Autodesk Inventor part; units mm, degrees
(part 2 of 2)
sketch "Sketch6" plane through (0.198, 6.7657, 76.2) normal (0.8660254, 0.5, 0) x (0, 0, -1)
  line L0 (9.5837, -3.7706) -> (68.3434, -3.7706) construction
  line L1 (68.3434, -3.7706) -> (68.3434, -8.4681) construction
  line L2 (68.3434, -8.4681) -> (9.5837, -8.4681) construction
  line L3 (9.5837, -8.4681) -> (9.5837, -3.7706) construction
  spline S0 degree 2 poles (10.7422, -7.0088) (10.4112, -7.0088) (9.9468, -6.8705) (9.7418, -6.7717) knots 0 0 0 1 2 2 2
  line L4 (9.7418, -6.7717) -> (9.7418, -6.2629)
  line L5 (9.7418, -6.2629) -> (9.7715, -6.2629)
  spline S1 degree 2 poles (9.7715, -6.2629) (9.9715, -6.4506) (10.4779, -6.6581) (10.7125, -6.6581) knots 0 0 0 1 2 2 2
  spline S2 degree 2 poles (10.7125, -6.6581) (11.0485, -6.6581) (11.3918, -6.379) (11.3918, -6.1492) knots 0 0 0 1 2 2 2
  spline S3 degree 2 poles (11.3918, -6.1492) (11.3918, -5.9665) (11.2115, -5.7392) (11.0164, -5.6824) knots 0 0 0 1 2 2 2
  spline S4 degree 2 poles (11.0164, -5.6824) (10.8756, -5.6429) (10.6409, -5.5886) (10.4655, -5.5441) knots 0 0 0 1 2 2 2
  spline S5 degree 2 poles (10.4655, -5.5441) (10.3075, -5.5021) (10.058, -5.3761) (9.9617, -5.2749) knots 0 0 0 1 2 2 2
  spline S6 degree 2 poles (9.9617, -5.2749) (9.8678, -5.1736) (9.7641, -4.9019) (9.7641, -4.724) knots 0 0 0 1 2 2 2
  spline S7 degree 2 poles (9.7641, -4.724) (9.7641, -4.3535) (10.342, -3.8521) (10.7891, -3.8521) knots 0 0 0 1 2 2 2
  spline S8 degree 2 poles (10.7891, -3.8521) (11.046, -3.8521) (11.5005, -3.9534) (11.6956, -4.0497) knots 0 0 0 1 2 2 2
  line L6 (11.6956, -4.0497) -> (11.6956, -4.5339)
  line L7 (11.6956, -4.5339) -> (11.666, -4.5339)
  spline S9 degree 2 poles (11.666, -4.5339) (11.5202, -4.4005) (11.0658, -4.2029) (10.8163, -4.2029) knots 0 0 0 1 2 2 2
  spline S10 degree 2 poles (10.8163, -4.2029) (10.5347, -4.2029) (10.1864, -4.4672) (10.1864, -4.6821) knots 0 0 0 1 2 2 2
  spline S11 degree 2 poles (10.1864, -4.6821) (10.1864, -4.8747) (10.3914, -5.1044) (10.5841, -5.1563) knots 0 0 0 1 2 2 2
  spline S12 degree 2 poles (10.5841, -5.1563) (10.7125, -5.1909) (11.0855, -5.2798) (11.209, -5.3169) knots 0 0 0 1 2 2 2
  spline S13 degree 2 poles (11.209, -5.3169) (11.5227, -5.4132) (11.8142, -5.801) (11.8142, -6.085) knots 0 0 0 1 2 2 2
  spline S14 degree 2 poles (11.8142, -6.085) (11.8142, -6.2653) (11.6684, -6.6111) (11.5375, -6.7322) knots 0 0 0 1 2 2 2
  spline S15 degree 2 poles (11.5375, -6.7322) (11.3918, -6.8656) (11.0213, -7.0088) (10.7422, -7.0088) knots 0 0 0 1 2 2 2
  spline S16 degree 2 poles (14.0767, -5.8109) (14.0767, -6.3888) (13.521, -7.0187) (13.0566, -7.0187) knots 0 0 0 1 2 2 2
  spline S17 degree 2 poles (13.0566, -7.0187) (12.5799, -7.0187) (12.034, -6.3691) (12.034, -5.8109) knots 0 0 0 1 2 2 2
  spline S18 degree 2 poles (12.034, -5.8109) (12.034, -5.2378) (12.5972, -4.603) (13.0566, -4.603) knots 0 0 0 1 2 2 2
  spline S19 degree 2 poles (13.0566, -4.603) (13.521, -4.603) (14.0767, -5.2353) (14.0767, -5.8109) knots 0 0 0 1 2 2 2
  spline S20 degree 2 poles (13.679, -5.8109) (13.679, -5.3663) (13.3555, -4.934) (13.0566, -4.934) knots 0 0 0 1 2 2 2
  spline S21 degree 2 poles (13.0566, -4.934) (12.7577, -4.934) (12.4317, -5.3663) (12.4317, -5.8109) knots 0 0 0 1 2 2 2
  spline S22 degree 2 poles (12.4317, -5.8109) (12.4317, -6.2431) (12.7577, -6.6877) (13.0566, -6.6877) knots 0 0 0 1 2 2 2
  spline S23 degree 2 poles (13.0566, -6.6877) (13.353, -6.6877) (13.679, -6.2505) (13.679, -5.8109) knots 0 0 0 1 2 2 2
  line L8 (17.0654, -6.9545) -> (17.0654, -5.6305)
  spline S24 degree 2 poles (17.0654, -5.6305) (17.0654, -5.4725) (17.0407, -5.2032) (17.0012, -5.1291) knots 0 0 0 1 2 2 2
  spline S25 degree 2 poles (17.0012, -5.1291) (16.9617, -5.0476) (16.811, -4.9686) (16.6801, -4.9686) knots 0 0 0 1 2 2 2
  spline S26 degree 2 poles (16.6801, -4.9686) (16.5615, -4.9686) (16.2898, -5.1143) (16.1466, -5.2526) knots 0 0 0 1 2 2 2
  spline S27 degree 2 poles (16.1466, -5.2526) (16.1491, -5.2872) (16.154, -5.3835) (16.154, -5.4478) knots 0 0 0 1 2 2 2
  line L9 (16.154, -5.4478) -> (16.154, -6.9545)
  line L10 (16.154, -6.9545) -> (15.7687, -6.9545)
  line L11 (15.7687, -6.9545) -> (15.7687, -5.6305)
  spline S28 degree 2 poles (15.7687, -5.6305) (15.7687, -5.4725) (15.744, -5.2032) (15.7044, -5.1291) knots 0 0 0 1 2 2 2
  spline S29 degree 2 poles (15.7044, -5.1291) (15.6649, -5.0476) (15.5143, -4.9686) (15.3833, -4.9686) knots 0 0 0 1 2 2 2
  spline S30 degree 2 poles (15.3833, -4.9686) (15.2598, -4.9686) (14.9857, -5.1242) (14.8572, -5.2452) knots 0 0 0 1 2 2 2
  line L12 (14.8572, -5.2452) -> (14.8572, -6.9545)
  line L13 (14.8572, -6.9545) -> (14.4719, -6.9545)
  line L14 (14.4719, -6.9545) -> (14.4719, -4.6672)
  line L15 (14.4719, -4.6672) -> (14.8572, -4.6672)
  line L16 (14.8572, -4.6672) -> (14.8572, -4.9192)
  spline S31 degree 2 poles (14.8572, -4.9192) (15.0079, -4.7685) (15.3043, -4.603) (15.4821, -4.603) knots 0 0 0 1 2 2 2
  spline S32 degree 2 poles (15.4821, -4.603) (15.6847, -4.603) (15.9984, -4.7883) (16.0799, -4.9982) knots 0 0 0 1 2 2 2
  spline S33 degree 2 poles (16.0799, -4.9982) (16.2553, -4.8031) (16.5862, -4.603) (16.7789, -4.603) knots 0 0 0 1 2 2 2
  spline S34 degree 2 poles (16.7789, -4.603) (16.9271, -4.603) (17.1692, -4.6944) (17.2581, -4.7981) knots 0 0 0 1 2 2 2
  spline S35 degree 2 poles (17.2581, -4.7981) (17.3495, -4.9019) (17.4507, -5.2131) (17.4507, -5.4478) knots 0 0 0 1 2 2 2
  line L17 (17.4507, -5.4478) -> (17.4507, -6.9545)
  line L18 (17.4507, -6.9545) -> (17.0654, -6.9545)
  spline S36 degree 2 poles (18.9846, -7.0063) (18.4363, -7.0063) (17.8336, -6.3913) (17.8336, -5.8232) knots 0 0 0 1 2 2 2
  spline S37 degree 2 poles (17.8336, -5.8232) (17.8336, -5.265) (18.419, -4.603) (18.8908, -4.603) knots 0 0 0 1 2 2 2
  spline S38 degree 2 poles (18.8908, -4.603) (19.1032, -4.603) (19.4317, -4.7265) (19.5527, -4.8574) knots 0 0 0 1 2 2 2
  spline S39 degree 2 poles (19.5527, -4.8574) (19.6762, -4.9883) (19.8071, -5.3663) (19.8071, -5.6404) knots 0 0 0 1 2 2 2
  line L19 (19.8071, -5.6404) -> (19.8071, -5.8504)
  line L20 (19.8071, -5.8504) -> (18.2239, -5.8504)
  spline S40 degree 2 poles (18.2239, -5.8504) (18.2239, -6.248) (18.624, -6.6704) (18.9797, -6.6704) knots 0 0 0 1 2 2 2
  spline S41 degree 2 poles (18.9797, -6.6704) (19.1057, -6.6704) (19.3502, -6.6136) (19.449, -6.5691) knots 0 0 0 1 2 2 2
  spline S42 degree 2 poles (19.449, -6.5691) (19.5527, -6.5197) (19.696, -6.4333) (19.7429, -6.3938) knots 0 0 0 1 2 2 2
  line L21 (19.7429, -6.3938) -> (19.7652, -6.3938)
  line L22 (19.7652, -6.3938) -> (19.7652, -6.8137)
  spline S43 degree 2 poles (19.7652, -6.8137) (19.6985, -6.8409) (19.4959, -6.9199) (19.4169, -6.9421) knots 0 0 0 1 2 2 2
  spline S44 degree 2 poles (19.4169, -6.9421) (19.3057, -6.9742) (19.123, -7.0063) (18.9846, -7.0063) knots 0 0 0 1 2 2 2
  spline S45 degree 2 poles (19.4317, -5.5564) (19.4268, -5.4008) (19.3625, -5.1736) (19.3008, -5.097) knots 0 0 0 1 2 2 2
  spline S46 degree 2 poles (19.3008, -5.097) (19.2341, -5.0106) (19.0241, -4.9192) (18.8685, -4.9192) knots 0 0 0 1 2 2 2
  spline S47 degree 2 poles (18.8685, -4.9192) (18.7154, -4.9192) (18.5005, -5.0106) (18.4116, -5.0995) knots 0 0 0 1 2 2 2
  spline S48 degree 2 poles (18.4116, -5.0995) (18.3251, -5.1909) (18.2362, -5.4107) (18.2239, -5.5564) knots 0 0 0 1 2 2 2
  line L23 (18.2239, -5.5564) -> (19.4317, -5.5564)
  line L24 (23.895, -6.9545) -> (23.3689, -6.9545)
  line L25 (23.3689, -6.9545) -> (22.4056, -5.7417)
  line L26 (22.4056, -5.7417) -> (21.9412, -5.7417)
  line L27 (21.9412, -5.7417) -> (21.9412, -6.9545)
  line L28 (21.9412, -6.9545) -> (21.5362, -6.9545)
  line L29 (21.5362, -6.9545) -> (21.5362, -3.9065)
  line L30 (21.5362, -3.9065) -> (22.3216, -3.9065)
  spline S49 degree 2 poles (22.3216, -3.9065) (22.5834, -3.9065) (22.9367, -3.9633) (23.0972, -4.067) knots 0 0 0 1 2 2 2
  spline S50 degree 2 poles (23.0972, -4.067) (23.2578, -4.1708) (23.443, -4.4943) (23.443, -4.7339) knots 0 0 0 1 2 2 2
  spline S51 degree 2 poles (23.443, -4.7339) (23.443, -5.0674) (23.1021, -5.5194) (22.8107, -5.6281) knots 0 0 0 1 2 2 2
  line L31 (22.8107, -5.6281) -> (23.895, -6.9545)
  spline S52 degree 2 poles (23.0206, -4.766) (23.0206, -4.6327) (22.9268, -4.4276) (22.828, -4.361) knots 0 0 0 1 2 2 2
  spline S53 degree 2 poles (22.828, -4.361) (22.7415, -4.3041) (22.5118, -4.2572) (22.3439, -4.2572) knots 0 0 0 1 2 2 2
  line L32 (22.3439, -4.2572) -> (21.9412, -4.2572)
  line L33 (21.9412, -4.2572) -> (21.9412, -5.4033)
  line L34 (21.9412, -5.4033) -> (22.2969, -5.4033)
  spline S54 degree 2 poles (22.2969, -5.4033) (22.4723, -5.4033) (22.7514, -5.3416) (22.8477, -5.2452) knots 0 0 0 1 2 2 2
  spline S55 degree 2 poles (22.8477, -5.2452) (22.9367, -5.1612) (23.0206, -4.9241) (23.0206, -4.766) knots 0 0 0 1 2 2 2
  spline S56 degree 2 poles (25.382, -6.7124) (25.335, -6.747) (25.177, -6.8705) (25.1029, -6.9075) knots 0 0 0 1 2 2 2
  spline S57 degree 2 poles (25.1029, -6.9075) (25.0016, -6.9619) (24.8114, -7.0187) (24.6385, -7.0187) knots 0 0 0 1 2 2 2
  spline S58 degree 2 poles (24.6385, -7.0187) (24.4977, -7.0187) (24.2433, -6.9125) (24.147, -6.8162) knots 0 0 0 1 2 2 2
  spline S59 degree 2 poles (24.147, -6.8162) (24.0556, -6.7223) (23.9444, -6.4456) (23.9444, -6.2925) knots 0 0 0 1 2 2 2
  spline S60 degree 2 poles (23.9444, -6.2925) (23.9444, -6.0554) (24.1445, -5.7195) (24.3619, -5.6231) knots 0 0 0 1 2 2 2
  spline S61 degree 2 poles (24.3619, -5.6231) (24.5545, -5.5342) (25.0782, -5.4675) (25.382, -5.4502) knots 0 0 0 1 2 2 2
  line L35 (25.382, -5.4502) -> (25.382, -5.3761)
  spline S62 degree 2 poles (25.382, -5.3761) (25.382, -5.2428) (25.3005, -5.0773) (25.2264, -5.0303) knots 0 0 0 1 2 2 2
  spline S63 degree 2 poles (25.2264, -5.0303) (25.1523, -4.9834) (24.9398, -4.9538) (24.8262, -4.9538) knots 0 0 0 1 2 2 2
  spline S64 degree 2 poles (24.8262, -4.9538) (24.6928, -4.9538) (24.3322, -5.0328) (24.1519, -5.1094) knots 0 0 0 1 2 2 2
  line L36 (24.1519, -5.1094) -> (24.1297, -5.1094)
  line L37 (24.1297, -5.1094) -> (24.1297, -4.7166)
  spline S65 degree 2 poles (24.1297, -4.7166) (24.2359, -4.687) (24.6336, -4.6129) (24.8287, -4.6129) knots 0 0 0 1 2 2 2
  spline S66 degree 2 poles (24.8287, -4.6129) (25.0658, -4.6129) (25.3894, -4.687) (25.5178, -4.7833) knots 0 0 0 1 2 2 2
  spline S67 degree 2 poles (25.5178, -4.7833) (25.6438, -4.8772) (25.7673, -5.1761) (25.7673, -5.391) knots 0 0 0 1 2 2 2
  line L38 (25.7673, -5.391) -> (25.7673, -6.9545)
  line L39 (25.7673, -6.9545) -> (25.382, -6.9545)
  line L40 (25.382, -6.9545) -> (25.382, -6.7124)
  line L41 (25.382, -6.3913) -> (25.382, -5.7565)
  spline S68 degree 2 poles (25.382, -5.7565) (25.2437, -5.7689) (24.8262, -5.8109) (24.6953, -5.8504) knots 0 0 0 1 2 2 2
  spline S69 degree 2 poles (24.6953, -5.8504) (24.5422, -5.8973) (24.3421, -6.0924) (24.3421, -6.2653) knots 0 0 0 1 2 2 2
  spline S70 degree 2 poles (24.3421, -6.2653) (24.3421, -6.4629) (24.5644, -6.663) (24.7768, -6.663) knots 0 0 0 1 2 2 2
  spline S71 degree 2 poles (24.7768, -6.663) (24.9571, -6.663) (25.2535, -6.5074) (25.382, -6.3913) knots 0 0 0 1 2 2 2
  line L42 (28.1039, -6.9545) -> (27.7186, -6.9545)
  line L43 (27.7186, -6.9545) -> (27.7186, -5.6503)
  spline S72 degree 2 poles (27.7186, -5.6503) (27.7186, -5.4922) (27.689, -5.2205) (27.6445, -5.139) knots 0 0 0 1 2 2 2
  spline S73 degree 2 poles (27.6445, -5.139) (27.5976, -5.0526) (27.4296, -4.9686) (27.2864, -4.9686) knots 0 0 0 1 2 2 2
  spline S74 degree 2 poles (27.2864, -4.9686) (27.1431, -4.9686) (26.8393, -5.1217) (26.6935, -5.2452) knots 0 0 0 1 2 2 2
  line L44 (26.6935, -5.2452) -> (26.6935, -6.9545)
  line L45 (26.6935, -6.9545) -> (26.3082, -6.9545)
  line L46 (26.3082, -6.9545) -> (26.3082, -4.6672)
  line L47 (26.3082, -4.6672) -> (26.6935, -4.6672)
  line L48 (26.6935, -4.6672) -> (26.6935, -4.9216)
  spline S75 degree 2 poles (26.6935, -4.9216) (26.8665, -4.766) (27.1999, -4.603) (27.3876, -4.603) knots 0 0 0 1 2 2 2
  spline S76 degree 2 poles (27.3876, -4.603) (27.7235, -4.603) (28.1039, -5.0476) (28.1039, -5.47) knots 0 0 0 1 2 2 2
  line L49 (28.1039, -5.47) -> (28.1039, -6.9545)
  line L50 (30.4035, -6.9545) -> (30.0182, -6.9545)
  line L51 (30.0182, -6.9545) -> (30.0182, -6.7223)
  spline S77 degree 2 poles (30.0182, -6.7223) (29.9293, -6.7964) (29.7984, -6.8952) (29.7094, -6.9372) knots 0 0 0 1 2 2 2
  spline S78 degree 2 poles (29.7094, -6.9372) (29.6279, -6.9767) (29.4526, -7.0187) (29.3365, -7.0187) knots 0 0 0 1 2 2 2
  spline S79 degree 2 poles (29.3365, -7.0187) (29.1487, -7.0187) (28.8326, -6.8631) (28.7214, -6.7124) knots 0 0 0 1 2 2 2
  spline S80 degree 2 poles (28.7214, -6.7124) (28.6103, -6.5617) (28.4868, -6.1171) (28.4868, -5.8281) knots 0 0 0 1 2 2 2
  spline S81 degree 2 poles (28.4868, -5.8281) (28.4868, -5.5268) (28.6424, -5.0871) (28.7782, -4.9216) knots 0 0 0 1 2 2 2
  spline S82 degree 2 poles (28.7782, -4.9216) (28.9042, -4.7734) (29.2574, -4.603) (29.4526, -4.603) knots 0 0 0 1 2 2 2
  spline S83 degree 2 poles (29.4526, -4.603) (29.623, -4.603) (29.8774, -4.6796) (30.0182, -4.7586) knots 0 0 0 1 2 2 2
  line L52 (30.0182, -4.7586) -> (30.0182, -3.7706)
  line L53 (30.0182, -3.7706) -> (30.4035, -3.7706)
  line L54 (30.4035, -3.7706) -> (30.4035, -6.9545)
  line L55 (30.0182, -6.3987) -> (30.0182, -5.0773)
  spline S84 degree 2 poles (30.0182, -5.0773) (29.8749, -5.0081) (29.6477, -4.9562) (29.5168, -4.9562) knots 0 0 0 1 2 2 2
  spline S85 degree 2 poles (29.5168, -4.9562) (29.2204, -4.9562) (28.8845, -5.4008) (28.8845, -5.8207) knots 0 0 0 1 2 2 2
  spline S86 degree 2 poles (28.8845, -5.8207) (28.8845, -6.2258) (29.1413, -6.6531) (29.4254, -6.6531) knots 0 0 0 1 2 2 2
  spline S87 degree 2 poles (29.4254, -6.6531) (29.5761, -6.6531) (29.8823, -6.5148) (30.0182, -6.3987) knots 0 0 0 1 2 2 2
  spline S88 degree 2 poles (32.8414, -5.8109) (32.8414, -6.3888) (32.2857, -7.0187) (31.8213, -7.0187) knots 0 0 0 1 2 2 2
  spline S89 degree 2 poles (31.8213, -7.0187) (31.3446, -7.0187) (30.7987, -6.3691) (30.7987, -5.8109) knots 0 0 0 1 2 2 2
  spline S90 degree 2 poles (30.7987, -5.8109) (30.7987, -5.2378) (31.3619, -4.603) (31.8213, -4.603) knots 0 0 0 1 2 2 2
  spline S91 degree 2 poles (31.8213, -4.603) (32.2857, -4.603) (32.8414, -5.2353) (32.8414, -5.8109) knots 0 0 0 1 2 2 2
  spline S92 degree 2 poles (32.4437, -5.8109) (32.4437, -5.3663) (32.1202, -4.934) (31.8213, -4.934) knots 0 0 0 1 2 2 2
  spline S93 degree 2 poles (31.8213, -4.934) (31.5224, -4.934) (31.1964, -5.3663) (31.1964, -5.8109) knots 0 0 0 1 2 2 2
  spline S94 degree 2 poles (31.1964, -5.8109) (31.1964, -6.2431) (31.5224, -6.6877) (31.8213, -6.6877) knots 0 0 0 1 2 2 2
  spline S95 degree 2 poles (31.8213, -6.6877) (32.1177, -6.6877) (32.4437, -6.2505) (32.4437, -5.8109) knots 0 0 0 1 2 2 2
  line L56 (35.8301, -6.9545) -> (35.8301, -5.6305)
  spline S96 degree 2 poles (35.8301, -5.6305) (35.8301, -5.4725) (35.8054, -5.2032) (35.7659, -5.1291) knots 0 0 0 1 2 2 2
  spline S97 degree 2 poles (35.7659, -5.1291) (35.7264, -5.0476) (35.5757, -4.9686) (35.4448, -4.9686) knots 0 0 0 1 2 2 2
  spline S98 degree 2 poles (35.4448, -4.9686) (35.3263, -4.9686) (35.0546, -5.1143) (34.9113, -5.2526) knots 0 0 0 1 2 2 2
  spline S99 degree 2 poles (34.9113, -5.2526) (34.9138, -5.2872) (34.9187, -5.3835) (34.9187, -5.4478) knots 0 0 0 1 2 2 2
  line L57 (34.9187, -5.4478) -> (34.9187, -6.9545)
  line L58 (34.9187, -6.9545) -> (34.5334, -6.9545)
  line L59 (34.5334, -6.9545) -> (34.5334, -5.6305)
  spline S100 degree 2 poles (34.5334, -5.6305) (34.5334, -5.4725) (34.5087, -5.2032) (34.4692, -5.1291) knots 0 0 0 1 2 2 2
  spline S101 degree 2 poles (34.4692, -5.1291) (34.4296, -5.0476) (34.279, -4.9686) (34.1481, -4.9686) knots 0 0 0 1 2 2 2
  spline S102 degree 2 poles (34.1481, -4.9686) (34.0246, -4.9686) (33.7504, -5.1242) (33.6219, -5.2452) knots 0 0 0 1 2 2 2
  line L60 (33.6219, -5.2452) -> (33.6219, -6.9545)
  line L61 (33.6219, -6.9545) -> (33.2366, -6.9545)
  line L62 (33.2366, -6.9545) -> (33.2366, -4.6672)
  line L63 (33.2366, -4.6672) -> (33.6219, -4.6672)
  line L64 (33.6219, -4.6672) -> (33.6219, -4.9192)
  spline S103 degree 2 poles (33.6219, -4.9192) (33.7726, -4.7685) (34.069, -4.603) (34.2469, -4.603) knots 0 0 0 1 2 2 2
  spline S104 degree 2 poles (34.2469, -4.603) (34.4494, -4.603) (34.7631, -4.7883) (34.8446, -4.9982) knots 0 0 0 1 2 2 2
  spline S105 degree 2 poles (34.8446, -4.9982) (35.02, -4.8031) (35.351, -4.603) (35.5436, -4.603) knots 0 0 0 1 2 2 2
  spline S106 degree 2 poles (35.5436, -4.603) (35.6918, -4.603) (35.9339, -4.6944) (36.0228, -4.7981) knots 0 0 0 1 2 2 2
  spline S107 degree 2 poles (36.0228, -4.7981) (36.1142, -4.9019) (36.2155, -5.2131) (36.2155, -5.4478) knots 0 0 0 1 2 2 2
  line L65 (36.2155, -5.4478) -> (36.2155, -6.9545)
  line L66 (36.2155, -6.9545) -> (35.8301, -6.9545)
  line L67 (38.8065, -6.9545) -> (38.8065, -4.2671)
  line L68 (38.8065, -4.2671) -> (37.7839, -4.2671)
  line L69 (37.7839, -4.2671) -> (37.7839, -3.9065)
  line L70 (37.7839, -3.9065) -> (40.2342, -3.9065)
  line L71 (40.2342, -3.9065) -> (40.2342, -4.2671)
  line L72 (40.2342, -4.2671) -> (39.2116, -4.2671)
  line L73 (39.2116, -4.2671) -> (39.2116, -6.9545)
  line L74 (39.2116, -6.9545) -> (38.8065, -6.9545)
  spline S108 degree 2 poles (41.5062, -7.0063) (40.9579, -7.0063) (40.3552, -6.3913) (40.3552, -5.8232) knots 0 0 0 1 2 2 2
  spline S109 degree 2 poles (40.3552, -5.8232) (40.3552, -5.265) (40.9406, -4.603) (41.4124, -4.603) knots 0 0 0 1 2 2 2
  spline S110 degree 2 poles (41.4124, -4.603) (41.6248, -4.603) (41.9533, -4.7265) (42.0743, -4.8574) knots 0 0 0 1 2 2 2
  spline S111 degree 2 poles (42.0743, -4.8574) (42.1978, -4.9883) (42.3288, -5.3663) (42.3288, -5.6404) knots 0 0 0 1 2 2 2
  line L75 (42.3288, -5.6404) -> (42.3288, -5.8504)
  line L76 (42.3288, -5.8504) -> (40.7455, -5.8504)
  spline S112 degree 2 poles (40.7455, -5.8504) (40.7455, -6.248) (41.1456, -6.6704) (41.5013, -6.6704) knots 0 0 0 1 2 2 2
  spline S113 degree 2 poles (41.5013, -6.6704) (41.6273, -6.6704) (41.8718, -6.6136) (41.9706, -6.5691) knots 0 0 0 1 2 2 2
  spline S114 degree 2 poles (41.9706, -6.5691) (42.0743, -6.5197) (42.2176, -6.4333) (42.2645, -6.3938) knots 0 0 0 1 2 2 2
  line L77 (42.2645, -6.3938) -> (42.2868, -6.3938)
  line L78 (42.2868, -6.3938) -> (42.2868, -6.8137)
  spline S115 degree 2 poles (42.2868, -6.8137) (42.2201, -6.8409) (42.0175, -6.9199) (41.9385, -6.9421) knots 0 0 0 1 2 2 2
  spline S116 degree 2 poles (41.9385, -6.9421) (41.8273, -6.9742) (41.6446, -7.0063) (41.5062, -7.0063) knots 0 0 0 1 2 2 2
  spline S117 degree 2 poles (41.9533, -5.5564) (41.9484, -5.4008) (41.8841, -5.1736) (41.8224, -5.097) knots 0 0 0 1 2 2 2
  spline S118 degree 2 poles (41.8224, -5.097) (41.7557, -5.0106) (41.5458, -4.9192) (41.3901, -4.9192) knots 0 0 0 1 2 2 2
  spline S119 degree 2 poles (41.3901, -4.9192) (41.237, -4.9192) (41.0221, -5.0106) (40.9332, -5.0995) knots 0 0 0 1 2 2 2
  spline S120 degree 2 poles (40.9332, -5.0995) (40.8467, -5.1909) (40.7578, -5.4107) (40.7455, -5.5564) knots 0 0 0 1 2 2 2
  line L79 (40.7455, -5.5564) -> (41.9533, -5.5564)
  spline S121 degree 2 poles (43.9935, -6.7124) (43.9466, -6.747) (43.7885, -6.8705) (43.7144, -6.9075) knots 0 0 0 1 2 2 2
  spline S122 degree 2 poles (43.7144, -6.9075) (43.6132, -6.9619) (43.423, -7.0187) (43.2501, -7.0187) knots 0 0 0 1 2 2 2
  spline S123 degree 2 poles (43.2501, -7.0187) (43.1093, -7.0187) (42.8549, -6.9125) (42.7585, -6.8162) knots 0 0 0 1 2 2 2
  spline S124 degree 2 poles (42.7585, -6.8162) (42.6671, -6.7223) (42.556, -6.4456) (42.556, -6.2925) knots 0 0 0 1 2 2 2
  spline S125 degree 2 poles (42.556, -6.2925) (42.556, -6.0554) (42.7561, -5.7195) (42.9734, -5.6231) knots 0 0 0 1 2 2 2
  spline S126 degree 2 poles (42.9734, -5.6231) (43.1661, -5.5342) (43.6897, -5.4675) (43.9935, -5.4502) knots 0 0 0 1 2 2 2
  line L80 (43.9935, -5.4502) -> (43.9935, -5.3761)
  spline S127 degree 2 poles (43.9935, -5.3761) (43.9935, -5.2428) (43.912, -5.0773) (43.8379, -5.0303) knots 0 0 0 1 2 2 2
  spline S128 degree 2 poles (43.8379, -5.0303) (43.7638, -4.9834) (43.5514, -4.9538) (43.4378, -4.9538) knots 0 0 0 1 2 2 2
  spline S129 degree 2 poles (43.4378, -4.9538) (43.3044, -4.9538) (42.9438, -5.0328) (42.7635, -5.1094) knots 0 0 0 1 2 2 2
  line L81 (42.7635, -5.1094) -> (42.7412, -5.1094)
  line L82 (42.7412, -5.1094) -> (42.7412, -4.7166)
  spline S130 degree 2 poles (42.7412, -4.7166) (42.8475, -4.687) (43.2451, -4.6129) (43.4403, -4.6129) knots 0 0 0 1 2 2 2
  spline S131 degree 2 poles (43.4403, -4.6129) (43.6774, -4.6129) (44.001, -4.687) (44.1294, -4.7833) knots 0 0 0 1 2 2 2
  spline S132 degree 2 poles (44.1294, -4.7833) (44.2554, -4.8772) (44.3789, -5.1761) (44.3789, -5.391) knots 0 0 0 1 2 2 2
  line L83 (44.3789, -5.391) -> (44.3789, -6.9545)
  line L84 (44.3789, -6.9545) -> (43.9935, -6.9545)
  line L85 (43.9935, -6.9545) -> (43.9935, -6.7124)
  line L86 (43.9935, -6.3913) -> (43.9935, -5.7565)
  spline S133 degree 2 poles (43.9935, -5.7565) (43.8552, -5.7689) (43.4378, -5.8109) (43.3069, -5.8504) knots 0 0 0 1 2 2 2
  spline S134 degree 2 poles (43.3069, -5.8504) (43.1537, -5.8973) (42.9537, -6.0924) (42.9537, -6.2653) knots 0 0 0 1 2 2 2
  spline S135 degree 2 poles (42.9537, -6.2653) (42.9537, -6.4629) (43.176, -6.663) (43.3884, -6.663) knots 0 0 0 1 2 2 2
  spline S136 degree 2 poles (43.3884, -6.663) (43.5687, -6.663) (43.8651, -6.5074) (43.9935, -6.3913) knots 0 0 0 1 2 2 2
  spline S137 degree 2 poles (45.8288, -7.0063) (45.5916, -7.0063) (45.1989, -6.8606) (45.0581, -6.7124) knots 0 0 0 1 2 2 2
  spline S138 degree 2 poles (45.0581, -6.7124) (44.9173, -6.5667) (44.7617, -6.1171) (44.7617, -5.8158) knots 0 0 0 1 2 2 2
  spline S139 degree 2 poles (44.7617, -5.8158) (44.7617, -5.5145) (44.9223, -5.0748) (45.0581, -4.9266) knots 0 0 0 1 2 2 2
  spline S140 degree 2 poles (45.0581, -4.9266) (45.194, -4.7759) (45.5966, -4.6154) (45.8288, -4.6154) knots 0 0 0 1 2 2 2
  spline S141 degree 2 poles (45.8288, -4.6154) (46.0165, -4.6154) (46.3672, -4.7216) (46.5031, -4.7907) knots 0 0 0 1 2 2 2
  line L87 (46.5031, -4.7907) -> (46.5031, -5.223)
  line L88 (46.5031, -5.223) -> (46.4809, -5.223)
  spline S142 degree 2 poles (46.4809, -5.223) (46.4389, -5.1884) (46.3104, -5.0995) (46.219, -5.0526) knots 0 0 0 1 2 2 2
  spline S143 degree 2 poles (46.219, -5.0526) (46.1375, -5.013) (45.9202, -4.9513) (45.8214, -4.9513) knots 0 0 0 1 2 2 2
  spline S144 degree 2 poles (45.8214, -4.9513) (45.5225, -4.9513) (45.1594, -5.4033) (45.1594, -5.8158) knots 0 0 0 1 2 2 2
  spline S145 degree 2 poles (45.1594, -5.8158) (45.1594, -6.2184) (45.5101, -6.6704) (45.8214, -6.6704) knots 0 0 0 1 2 2 2
  spline S146 degree 2 poles (45.8214, -6.6704) (46.0091, -6.6704) (46.3499, -6.5148) (46.4809, -6.3938) knots 0 0 0 1 2 2 2
  line L89 (46.4809, -6.3938) -> (46.5031, -6.3938)
  line L90 (46.5031, -6.3938) -> (46.5031, -6.826)
  spline S147 degree 2 poles (46.5031, -6.826) (46.4463, -6.8532) (46.2734, -6.9298) (46.2042, -6.9471) knots 0 0 0 1 2 2 2
  spline S148 degree 2 poles (46.2042, -6.9471) (46.1054, -6.9767) (45.9498, -7.0063) (45.8288, -7.0063) knots 0 0 0 1 2 2 2
  line L91 (48.6495, -6.9545) -> (48.2642, -6.9545)
  line L92 (48.2642, -6.9545) -> (48.2642, -5.6503)
  spline S149 degree 2 poles (48.2642, -5.6503) (48.2642, -5.4922) (48.2346, -5.2205) (48.1901, -5.139) knots 0 0 0 1 2 2 2
  spline S150 degree 2 poles (48.1901, -5.139) (48.1432, -5.0526) (47.9752, -4.9686) (47.8319, -4.9686) knots 0 0 0 1 2 2 2
  spline S151 degree 2 poles (47.8319, -4.9686) (47.6887, -4.9686) (47.3849, -5.1217) (47.2391, -5.2452) knots 0 0 0 1 2 2 2
  line L93 (47.2391, -5.2452) -> (47.2391, -6.9545)
  line L94 (47.2391, -6.9545) -> (46.8538, -6.9545)
  line L95 (46.8538, -6.9545) -> (46.8538, -3.7706)
  line L96 (46.8538, -3.7706) -> (47.2391, -3.7706)
  line L97 (47.2391, -3.7706) -> (47.2391, -4.9216)
  spline S152 degree 2 poles (47.2391, -4.9216) (47.412, -4.766) (47.7455, -4.603) (47.9332, -4.603) knots 0 0 0 1 2 2 2
  spline S153 degree 2 poles (47.9332, -4.603) (48.2691, -4.603) (48.6495, -5.0476) (48.6495, -5.47) knots 0 0 0 1 2 2 2
  line L98 (48.6495, -5.47) -> (48.6495, -6.9545)
  spline S154 degree 2 poles (50.1834, -7.0063) (49.6351, -7.0063) (49.0324, -6.3913) (49.0324, -5.8232) knots 0 0 0 1 2 2 2
  spline S155 degree 2 poles (49.0324, -5.8232) (49.0324, -5.265) (49.6178, -4.603) (50.0895, -4.603) knots 0 0 0 1 2 2 2
  spline S156 degree 2 poles (50.0895, -4.603) (50.302, -4.603) (50.6305, -4.7265) (50.7515, -4.8574) knots 0 0 0 1 2 2 2
  spline S157 degree 2 poles (50.7515, -4.8574) (50.875, -4.9883) (51.0059, -5.3663) (51.0059, -5.6404) knots 0 0 0 1 2 2 2
  line L99 (51.0059, -5.6404) -> (51.0059, -5.8504)
  line L100 (51.0059, -5.8504) -> (49.4226, -5.8504)
  spline S158 degree 2 poles (49.4226, -5.8504) (49.4226, -6.248) (49.8228, -6.6704) (50.1785, -6.6704) knots 0 0 0 1 2 2 2
  spline S159 degree 2 poles (50.1785, -6.6704) (50.3044, -6.6704) (50.549, -6.6136) (50.6478, -6.5691) knots 0 0 0 1 2 2 2
  spline S160 degree 2 poles (50.6478, -6.5691) (50.7515, -6.5197) (50.8948, -6.4333) (50.9417, -6.3938) knots 0 0 0 1 2 2 2
  line L101 (50.9417, -6.3938) -> (50.9639, -6.3938)
  line L102 (50.9639, -6.3938) -> (50.9639, -6.8137)
  spline S161 degree 2 poles (50.9639, -6.8137) (50.8972, -6.8409) (50.6947, -6.9199) (50.6157, -6.9421) knots 0 0 0 1 2 2 2
  spline S162 degree 2 poles (50.6157, -6.9421) (50.5045, -6.9742) (50.3217, -7.0063) (50.1834, -7.0063) knots 0 0 0 1 2 2 2
  spline S163 degree 2 poles (50.6305, -5.5564) (50.6255, -5.4008) (50.5613, -5.1736) (50.4996, -5.097) knots 0 0 0 1 2 2 2
  spline S164 degree 2 poles (50.4996, -5.097) (50.4329, -5.0106) (50.2229, -4.9192) (50.0673, -4.9192) knots 0 0 0 1 2 2 2
  spline S165 degree 2 poles (50.0673, -4.9192) (49.9142, -4.9192) (49.6993, -5.0106) (49.6104, -5.0995) knots 0 0 0 1 2 2 2
  spline S166 degree 2 poles (49.6104, -5.0995) (49.5239, -5.1909) (49.435, -5.4107) (49.4226, -5.5564) knots 0 0 0 1 2 2 2
  line L103 (49.4226, -5.5564) -> (50.6305, -5.5564)
  line L104 (52.609, -5.0797) -> (52.5892, -5.0797)
  spline S167 degree 2 poles (52.5892, -5.0797) (52.5447, -5.0674) (52.4484, -5.0624) (52.3817, -5.0624) knots 0 0 0 1 2 2 2
  spline S168 degree 2 poles (52.3817, -5.0624) (52.2261, -5.0624) (51.9198, -5.1983) (51.7815, -5.3317) knots 0 0 0 1 2 2 2
  line L105 (51.7815, -5.3317) -> (51.7815, -6.9545)
  line L106 (51.7815, -6.9545) -> (51.3962, -6.9545)
  line L107 (51.3962, -6.9545) -> (51.3962, -4.6672)
  line L108 (51.3962, -4.6672) -> (51.7815, -4.6672)
  line L109 (51.7815, -4.6672) -> (51.7815, -5.0081)
  spline S169 degree 2 poles (51.7815, -5.0081) (51.9915, -4.8204) (52.3051, -4.6672) (52.4533, -4.6672) knots 0 0 0 1 2 2 2
  spline S170 degree 2 poles (52.4533, -4.6672) (52.5126, -4.6672) (52.5719, -4.6722) (52.609, -4.6796) knots 0 0 0 1 2 2 2
  line L110 (52.609, -4.6796) -> (52.609, -5.0797)
  spline S171 degree 2 poles (53.5253, -7.0088) (53.2956, -7.0088) (52.898, -6.8853) (52.767, -6.8162) knots 0 0 0 1 2 2 2
  line L111 (52.767, -6.8162) -> (52.767, -6.3839)
  line L112 (52.767, -6.3839) -> (52.7868, -6.3839)
  spline S172 degree 2 poles (52.7868, -6.3839) (52.8362, -6.4234) (52.9696, -6.5173) (53.0807, -6.5691) knots 0 0 0 1 2 2 2
  spline S173 degree 2 poles (53.0807, -6.5691) (53.1771, -6.6161) (53.4142, -6.6852) (53.5402, -6.6852) knots 0 0 0 1 2 2 2
  spline S174 degree 2 poles (53.5402, -6.6852) (53.6315, -6.6852) (53.8415, -6.6432) (53.8909, -6.6087) knots 0 0 0 1 2 2 2
  spline S175 degree 2 poles (53.8909, -6.6087) (53.9625, -6.5617) (54.0267, -6.4555) (54.0267, -6.3468) knots 0 0 0 1 2 2 2
  spline S176 degree 2 poles (54.0267, -6.3468) (54.0267, -6.211) (53.8785, -6.0702) (53.6884, -6.0233) knots 0 0 0 1 2 2 2
  spline S177 degree 2 poles (53.6884, -6.0233) (53.6143, -6.006) (53.3771, -5.9566) (53.2759, -5.9294) knots 0 0 0 1 2 2 2
  spline S178 degree 2 poles (53.2759, -5.9294) (53.014, -5.8528) (52.7769, -5.5367) (52.7769, -5.3119) knots 0 0 0 1 2 2 2
  spline S179 degree 2 poles (52.7769, -5.3119) (52.7769, -5.0007) (53.2438, -4.6129) (53.6291, -4.6129) knots 0 0 0 1 2 2 2
  spline S180 degree 2 poles (53.6291, -4.6129) (53.8193, -4.6129) (54.2046, -4.7068) (54.3355, -4.7784) knots 0 0 0 1 2 2 2
  line L113 (54.3355, -4.7784) -> (54.3355, -5.1909)
  line L114 (54.3355, -5.1909) -> (54.3157, -5.1909)
  spline S181 degree 2 poles (54.3157, -5.1909) (54.1675, -5.0723) (53.8069, -4.9365) (53.6217, -4.9365) knots 0 0 0 1 2 2 2
  spline S182 degree 2 poles (53.6217, -4.9365) (53.4315, -4.9365) (53.1697, -5.097) (53.1697, -5.2576) knots 0 0 0 1 2 2 2
  spline S183 degree 2 poles (53.1697, -5.2576) (53.1697, -5.4033) (53.3253, -5.5441) (53.4982, -5.5886) knots 0 0 0 1 2 2 2
  spline S184 degree 2 poles (53.4982, -5.5886) (53.5821, -5.6108) (53.7946, -5.6552) (53.9107, -5.6824) knots 0 0 0 1 2 2 2
  spline S185 degree 2 poles (53.9107, -5.6824) (54.1626, -5.7466) (54.4195, -6.0406) (54.4195, -6.295) knots 0 0 0 1 2 2 2
  spline S186 degree 2 poles (54.4195, -6.295) (54.4195, -6.4432) (54.3034, -6.705) (54.1898, -6.8013) knots 0 0 0 1 2 2 2
  spline S187 degree 2 poles (54.1898, -6.8013) (54.0687, -6.9026) (53.76, -7.0088) (53.5253, -7.0088) knots 0 0 0 1 2 2 2
  line L115 (58.2974, -6.9545) -> (57.8429, -6.9545)
  line L116 (57.8429, -6.9545) -> (56.4943, -4.3264)
  line L117 (56.4943, -4.3264) -> (56.4943, -6.9545)
  line L118 (56.4943, -6.9545) -> (56.1164, -6.9545)
  line L119 (56.1164, -6.9545) -> (56.1164, -3.9065)
  line L120 (56.1164, -3.9065) -> (56.6919, -3.9065)
  line L121 (56.6919, -3.9065) -> (57.9195, -6.3197)
  line L122 (57.9195, -6.3197) -> (57.9195, -3.9065)
  line L123 (57.9195, -3.9065) -> (58.2974, -3.9065)
  line L124 (58.2974, -3.9065) -> (58.2974, -6.9545)
  spline S188 degree 2 poles (60.1598, -6.7124) (60.1129, -6.747) (59.9548, -6.8705) (59.8807, -6.9075) knots 0 0 0 1 2 2 2
  spline S189 degree 2 poles (59.8807, -6.9075) (59.7794, -6.9619) (59.5892, -7.0187) (59.4163, -7.0187) knots 0 0 0 1 2 2 2
  spline S190 degree 2 poles (59.4163, -7.0187) (59.2755, -7.0187) (59.0211, -6.9125) (58.9248, -6.8162) knots 0 0 0 1 2 2 2
  spline S191 degree 2 poles (58.9248, -6.8162) (58.8334, -6.7223) (58.7223, -6.4456) (58.7223, -6.2925) knots 0 0 0 1 2 2 2
  spline S192 degree 2 poles (58.7223, -6.2925) (58.7223, -6.0554) (58.9223, -5.7195) (59.1397, -5.6231) knots 0 0 0 1 2 2 2
  spline S193 degree 2 poles (59.1397, -5.6231) (59.3323, -5.5342) (59.856, -5.4675) (60.1598, -5.4502) knots 0 0 0 1 2 2 2
  line L125 (60.1598, -5.4502) -> (60.1598, -5.3761)
  spline S194 degree 2 poles (60.1598, -5.3761) (60.1598, -5.2428) (60.0783, -5.0773) (60.0042, -5.0303) knots 0 0 0 1 2 2 2
  spline S195 degree 2 poles (60.0042, -5.0303) (59.9301, -4.9834) (59.7177, -4.9538) (59.604, -4.9538) knots 0 0 0 1 2 2 2
  spline S196 degree 2 poles (59.604, -4.9538) (59.4707, -4.9538) (59.11, -5.0328) (58.9297, -5.1094) knots 0 0 0 1 2 2 2
  line L126 (58.9297, -5.1094) -> (58.9075, -5.1094)
  line L127 (58.9075, -5.1094) -> (58.9075, -4.7166)
  spline S197 degree 2 poles (58.9075, -4.7166) (59.0137, -4.687) (59.4114, -4.6129) (59.6065, -4.6129) knots 0 0 0 1 2 2 2
  spline S198 degree 2 poles (59.6065, -4.6129) (59.8436, -4.6129) (60.1672, -4.687) (60.2957, -4.7833) knots 0 0 0 1 2 2 2
  spline S199 degree 2 poles (60.2957, -4.7833) (60.4216, -4.8772) (60.5451, -5.1761) (60.5451, -5.391) knots 0 0 0 1 2 2 2
  line L128 (60.5451, -5.391) -> (60.5451, -6.9545)
  line L129 (60.5451, -6.9545) -> (60.1598, -6.9545)
  line L130 (60.1598, -6.9545) -> (60.1598, -6.7124)
  line L131 (60.1598, -6.3913) -> (60.1598, -5.7565)
  spline S200 degree 2 poles (60.1598, -5.7565) (60.0215, -5.7689) (59.604, -5.8109) (59.4731, -5.8504) knots 0 0 0 1 2 2 2
  spline S201 degree 2 poles (59.4731, -5.8504) (59.32, -5.8973) (59.1199, -6.0924) (59.1199, -6.2653) knots 0 0 0 1 2 2 2
  spline S202 degree 2 poles (59.1199, -6.2653) (59.1199, -6.4629) (59.3422, -6.663) (59.5546, -6.663) knots 0 0 0 1 2 2 2
  spline S203 degree 2 poles (59.5546, -6.663) (59.735, -6.663) (60.0314, -6.5074) (60.1598, -6.3913) knots 0 0 0 1 2 2 2
  line L132 (63.6796, -6.9545) -> (63.6796, -5.6305)
  spline S204 degree 2 poles (63.6796, -5.6305) (63.6796, -5.4725) (63.6549, -5.2032) (63.6154, -5.1291) knots 0 0 0 1 2 2 2
  spline S205 degree 2 poles (63.6154, -5.1291) (63.5758, -5.0476) (63.4252, -4.9686) (63.2943, -4.9686) knots 0 0 0 1 2 2 2
  spline S206 degree 2 poles (63.2943, -4.9686) (63.1757, -4.9686) (62.904, -5.1143) (62.7607, -5.2526) knots 0 0 0 1 2 2 2
  spline S207 degree 2 poles (62.7607, -5.2526) (62.7632, -5.2872) (62.7681, -5.3835) (62.7681, -5.4478) knots 0 0 0 1 2 2 2
  line L133 (62.7681, -5.4478) -> (62.7681, -6.9545)
  line L134 (62.7681, -6.9545) -> (62.3828, -6.9545)
  line L135 (62.3828, -6.9545) -> (62.3828, -5.6305)
  spline S208 degree 2 poles (62.3828, -5.6305) (62.3828, -5.4725) (62.3581, -5.2032) (62.3186, -5.1291) knots 0 0 0 1 2 2 2
  spline S209 degree 2 poles (62.3186, -5.1291) (62.2791, -5.0476) (62.1284, -4.9686) (61.9975, -4.9686) knots 0 0 0 1 2 2 2
  spline S210 degree 2 poles (61.9975, -4.9686) (61.874, -4.9686) (61.5998, -5.1242) (61.4714, -5.2452) knots 0 0 0 1 2 2 2
  line L136 (61.4714, -5.2452) -> (61.4714, -6.9545)
  line L137 (61.4714, -6.9545) -> (61.0861, -6.9545)
  line L138 (61.0861, -6.9545) -> (61.0861, -4.6672)
  line L139 (61.0861, -4.6672) -> (61.4714, -4.6672)
  line L140 (61.4714, -4.6672) -> (61.4714, -4.9192)
  spline S211 degree 2 poles (61.4714, -4.9192) (61.622, -4.7685) (61.9185, -4.603) (62.0963, -4.603) knots 0 0 0 1 2 2 2
  spline S212 degree 2 poles (62.0963, -4.603) (62.2988, -4.603) (62.6125, -4.7883) (62.694, -4.9982) knots 0 0 0 1 2 2 2
  spline S213 degree 2 poles (62.694, -4.9982) (62.8694, -4.8031) (63.2004, -4.603) (63.3931, -4.603) knots 0 0 0 1 2 2 2
  spline S214 degree 2 poles (63.3931, -4.603) (63.5413, -4.603) (63.7833, -4.6944) (63.8722, -4.7981) knots 0 0 0 1 2 2 2
  spline S215 degree 2 poles (63.8722, -4.7981) (63.9636, -4.9019) (64.0649, -5.2131) (64.0649, -5.4478) knots 0 0 0 1 2 2 2
  line L141 (64.0649, -5.4478) -> (64.0649, -6.9545)
  line L142 (64.0649, -6.9545) -> (63.6796, -6.9545)
  spline S216 degree 2 poles (65.5988, -7.0063) (65.0504, -7.0063) (64.4477, -6.3913) (64.4477, -5.8232) knots 0 0 0 1 2 2 2
  spline S217 degree 2 poles (64.4477, -5.8232) (64.4477, -5.265) (65.0331, -4.603) (65.5049, -4.603) knots 0 0 0 1 2 2 2
  spline S218 degree 2 poles (65.5049, -4.603) (65.7173, -4.603) (66.0458, -4.7265) (66.1669, -4.8574) knots 0 0 0 1 2 2 2
  spline S219 degree 2 poles (66.1669, -4.8574) (66.2904, -4.9883) (66.4213, -5.3663) (66.4213, -5.6404) knots 0 0 0 1 2 2 2
  line L143 (66.4213, -5.6404) -> (66.4213, -5.8504)
  line L144 (66.4213, -5.8504) -> (64.838, -5.8504)
  spline S220 degree 2 poles (64.838, -5.8504) (64.838, -6.248) (65.2382, -6.6704) (65.5938, -6.6704) knots 0 0 0 1 2 2 2
  spline S221 degree 2 poles (65.5938, -6.6704) (65.7198, -6.6704) (65.9643, -6.6136) (66.0631, -6.5691) knots 0 0 0 1 2 2 2
  spline S222 degree 2 poles (66.0631, -6.5691) (66.1669, -6.5197) (66.3101, -6.4333) (66.3571, -6.3938) knots 0 0 0 1 2 2 2
  line L145 (66.3571, -6.3938) -> (66.3793, -6.3938)
  line L146 (66.3793, -6.3938) -> (66.3793, -6.8137)
  spline S223 degree 2 poles (66.3793, -6.8137) (66.3126, -6.8409) (66.1101, -6.9199) (66.031, -6.9421) knots 0 0 0 1 2 2 2
  spline S224 degree 2 poles (66.031, -6.9421) (65.9199, -6.9742) (65.7371, -7.0063) (65.5988, -7.0063) knots 0 0 0 1 2 2 2
  spline S225 degree 2 poles (66.0458, -5.5564) (66.0409, -5.4008) (65.9767, -5.1736) (65.9149, -5.097) knots 0 0 0 1 2 2 2
  spline S226 degree 2 poles (65.9149, -5.097) (65.8482, -5.0106) (65.6383, -4.9192) (65.4827, -4.9192) knots 0 0 0 1 2 2 2
  spline S227 degree 2 poles (65.4827, -4.9192) (65.3295, -4.9192) (65.1147, -5.0106) (65.0257, -5.0995) knots 0 0 0 1 2 2 2
  spline S228 degree 2 poles (65.0257, -5.0995) (64.9393, -5.1909) (64.8504, -5.4107) (64.838, -5.5564) knots 0 0 0 1 2 2 2
  line L147 (64.838, -5.5564) -> (66.0458, -5.5564)
  point P0 (76.2, -5.7603)
  point P1 (0, 5.7603)
  constraints: 2 other
extrude "Extrusion5" add sketch "Sketch6" along normal blind 0.2286
body "Solid1"
